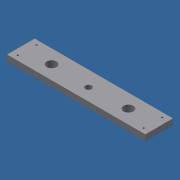
# Autodesk Inventor part: PlateHeatbed
Saved by Autodesk Inventor 2018 (Build 220112000, 112)
## iProperties
Created: 2022-08-31
Part Number: PlateHeatbed
Material: Generic
Document SubType Name: Modeling
Designer: Nathann
Density: 1 g/cm^3
Appearance: Default
Author: Nathann
Autodesk Inventor part; units mm, degrees
ref_plane "YZ Plane" through (0, 0, 0) normal (1, 0, 0) x (0, 1, 0)
ref_plane "XZ Plane" through (0, 0, 0) normal (0, 1, 0) x (-1, 0, 0)
ref_plane "XY Plane" through (0, 0, 0) normal (0, 0, 1) x (1, 0, 0)
sketch "Sketch1" plane through (0, 0, 0) normal (0, 0, 1) x (1, 0, 0)
  line L0 (0, 0) -> (-225, 0)
  line L1 (-225, 0) -> (-225, 45)
  line L2 (-225, 45) -> (0, 45)
  line L3 (0, 45) -> (0, 0)
  circle A0 centre (-10, 37.5) radius 1.5
  circle A1 centre (-10, 7.5) radius 1.5
  circle A2 centre (-214.479, 37.5) radius 1.5
  circle A3 centre (-215, 7.5) radius 1.5
  circle A4 centre (-112.5, 20) radius 5.1
  circle A5 centre (-175, 22.5) radius 8
  circle A6 centre (-50, 22.5) radius 8
  dimension "d0" = 45
  dimension "d1" = 225
  dimension "d2" = 30
  dimension "d3" = 3
  dimension "d4" = 3
  dimension "d5" = 7.5
  dimension "d6" = 7.5
  dimension "d7" = 3
  dimension "d8" = 3
  dimension "d9" = 30
  dimension "d10" = 10
  dimension "d11" = 10
  dimension "d14" = 16
  dimension "d15" = 16
  dimension "d16" = 22.5
  dimension "d17" = 22.5
  dimension "d18" = 50
  dimension "d19" = 50
  dimension "d20" = 10.2
  dimension "d21" = 25
  dimension "d22" = 112.5
  constraints: 8 end point, 7 centre point, 2 parallel, 1 horizontal, 1 perpendicular
  measures "d0" distance of L2.end L0.start
  measures "d1" distance of L1.end L2.end
  measures "d2" distance of A1.centre A0.centre
  measures "d3" diameter of A0
  measures "d4" diameter of A1
  measures "d5" distance from line of L0 A1.centre
  measures "d6" distance from line of L0 A3.centre
  measures "d7" diameter of A3
  measures "d8" diameter of A2
  measures "d9" vertical distance of A3.centre A2.centre
  measures "d10" distance from line of L1 A3.centre
  measures "d11" distance from line of L3 A1.centre
  measures "d14" diameter of A6
  measures "d15" diameter of A5
  measures "d16" distance from line of L0 A5.centre
  measures "d17" distance from line of L0 A6.centre
  measures "d18" distance from line of L3 A6.centre
  measures "d19" distance from line of L1 A5.centre
  measures "d20" diameter of A4
  measures "d21" distance from line of L2 A4.centre
  measures "d22" distance from line of L1 A4.centre
extrude "Extrusion1" add sketch "Sketch1" along normal blind 10
equation "\"d6\" = d5"
equation "\"d7\" = d4"
equation "\"d8\" = d7"
equation "\"d9\" = d2"
equation "\"d16\" = 0.5 * d0"
equation "\"d17\" = 0.5 * d0"
equation "\"d22\" = 0.5 * d1"
body "Solid1"
